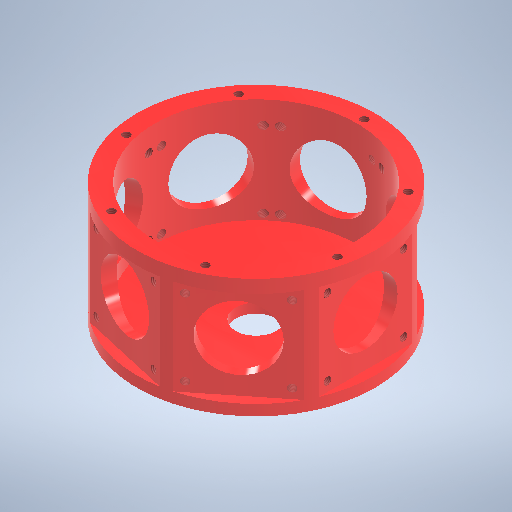
# Autodesk Inventor part: Gehäuse
Saved by Autodesk Inventor 2025 (Build 290162010, 162A)
## iProperties
Created: 2024-03-07
Part Number: Gehäuse
Material: Aluminum 6061
Document SubType Name: Modeling
Designer: ffogue
Density: 2.7 g/cm^3
Appearance: Light Red
Author: ffogue
Autodesk Inventor part; units mm, degrees
ref_plane "XZ Plane" through (0, 0, 0) normal (0, 1, 0) x (-1, 0, 0)
ref_plane "XY Plane" through (0, 0, 0) normal (0, 0, 1) x (1, 0, 0)
sketch "Skizze1" plane through (0, 0, 0) normal (0, 0, 1) x (1, 0, 0)
  circle A0 centre (0, 0) radius 50
  dimension "d0" = 100
  constraints: 1 centre point, 1 coincident
  measures "d0" diameter of A0
extrude "Extrusion1" add sketch "Skizze1" against normal blind 50
ref_plane "Arbeitsebene1" through (50, 0, 0) normal (1, 0, 0) x (0, 1, 0)
sketch "Skizze2" plane through (50, 0, 0) normal (1, 0, 0) x (0, 1, 0)
  line L0 (0, 0) -> (0, -28.5923) construction
  line L1 (-50, 0) -> (-50, -50) projected
  line L2 (-20, -5.5) -> (20, -5.5)
  line L3 (20, -5.5) -> (20, -45.5)
  line L4 (20, -45.5) -> (-20, -45.5)
  line L5 (-20, -45.5) -> (-20, -5.5)
  line L6 (-50, -50) -> (50, -50) construction
  dimension "d5" = 40
  dimension "d6" = 40
  dimension "d76" = 4.5
  constraints: 10 end point, 2 parallel, 1 horizontal, 1 perpendicular, 1 vertical, 1 other
  measures "d5" distance between parallel lines of L3 L5
  measures "d6" distance between parallel lines of L4 L2
  measures "d76" distance between parallel lines of L6 L4
extrude "Extrusion2" cut sketch "Skizze2" against normal blind 4
pattern_circular "Runde Anordnung1" count 7 over 360 about axis through (0, 0, 0) along (0, 0, -1) of "Extrusion2"
sketch "Skizze6" plane through (0, 0, -50) normal (0, 0, -1) x (-1, 0, 0)
  circle A0 centre (0, 0) radius 42.5
  circle A1 centre (0, 0) radius 40
  dimension "d25" = 85
  dimension "d26" = 80
  constraints: 2 centre point, 2 coincident
  measures "d25" diameter of A0
  measures "d26" diameter of A1
extrude "Extrusion9" cut sketch "Skizze6" against normal blind 4 contours A1
extrude "Extrusion10" add sketch "Skizze6" along normal blind 4
sketch "Sketch20" plane through (0, 0, -46) normal (0, 0, -1) x (-1, 0, 0)
  circle A0 centre (0, 0) radius 21.5
  dimension "d85" = 43
  constraints: 1 centre point, 1 coincident
  measures "d85" diameter of A0
extrude "Extrusion11" add sketch "Sketch20" along normal up to surface (8 mm away)
sketch "Sketch21" plane through (0, 0, -54) normal (0, 0, -1) x (-1, 0, 0)
  circle A0 centre (0, 0) radius 21.5 construction
  constraints: 1 coincident
hole "Hole5" at (0, 0, -54) direction (0, 0, 1) diameter 17.1 depth 4
sketch "Sketch22" plane through (0, 0, 0) normal (0, 0, 1) x (1, 0, 0)
  circle A0 centre (0, 0) radius 50 construction
  constraints: 1 coincident
hole "Hole6" at (0, 0, 0) direction (0, 0, -1) diameter 85 depth 44
sketch "Sketch24" plane through (0, 0, -50) normal (0, 0, -1) x (-1, 0, 0)
  circle A0 centre (0, 0) radius 21.5 construction
  constraints: 1 coincident
hole "Hole7" at (0, 0, -50) direction (0, 0, 1) diameter 35 depth 11
sketch "Sketch25" plane through (-32.9422, 37.614, -5.5) normal (-0.9009689, 0.4338837, 0) x (0.4338837, 0.9009689, 0)
  line L0 (0, 40) -> (-39.1918, 40) construction
  line L1 (0, 40) -> (0, 0) construction
  point P0 (-19.5959, -5.5)
  point P1 (-35.5959, 36)
  point P2 (-3.5959, 36)
  point P3 (-35.5959, 4)
  point P4 (-3.5959, 4)
  point P5 (-19.5959, 40)
  point P6 (0, 20)
  dimension "d111" = 32
  dimension "d112" = 32
  dimension "d113" = 16
  dimension "d114" = 16
  constraints: 2 horizontal alignment, 2 midpoint, 2 vertical alignment
  measures "d111" distance of point (-3.596, 36) point (-35.596, 36)
  measures "d112" distance of point (-35.596, 4) point (-35.596, 36)
  measures "d113" horizontal distance of point (-19.596, 40) point (-35.596, 36)
  measures "d114" vertical distance of point (0, 20) point (-3.596, 36)
hole "Hole8" at (-48.3867, 5.5432, -41.5) at (-34.5024, 34.3742, -41.5) at (-48.3867, 5.5432, -9.5) at (-34.5024, 34.3742, -9.5) direction (0.9009689, -0.4338837, 0) diameter 3.242 depth 10 tip angle 118 thread size "M4x0.7" class "6H" standard "ISO Metric profile"
pattern_circular "Circular Pattern4" count 7 over 360 about axis through (0, 0, -50) along (0, 0, 1) of "Hole8"
sketch "Sketch27" plane through (13.3598, -48.1821, -45.5) normal (0.6234898, -0.7818315, 0) x (0.7818315, 0.6234898, 0)
  circle A0 centre (19.5959, 21) radius 13.5
  line L0 (0, 0) -> (0, 40) construction
  line L1 (-22.9041, -8.5) -> (62.0959, -8.5) construction
  line L2 (0, 40) -> (39.1918, 40) construction
  line L3 (69.5959, 45.5) -> (-30.4041, 45.5) construction
  point P0 (19.5959, 45.5)
  point P1 (0, 20)
  point P2 (19.5959, 40)
  dimension "d132" = 27
  dimension "d153" = 24.5
  constraints: 2 midpoint, 1 centre point, 1 vertical alignment
  measures "d132" diameter of A0
  measures "d153" distance from line of L3 A0.centre
extrude "Extrusion12" cut sketch "Sketch27" against normal up to surface
pattern_circular "Circular Pattern5" count 7 over 360 about axis through (0, 0, -22) along (0, 0, 1) of "Extrusion12"
sketch "Sketch31" plane through (0, 0, -50) normal (0, 0, -1) x (-1, 0, 0)
  circle A0 centre (0, 0) radius 46 construction
  point P0 (0, 46)
  dimension "d142" = 92
  constraints: 2 vertical alignment, 1 coincident, 2 other
hole "Hole10" at (0, 46, -50) direction (0, 0, 1) diameter 4 depth 4
pattern_circular "Circular Pattern6" count 7 over 360 about axis through (0, 0, -50) along (0, 0, -1) of "Hole10"
sketch "Sketch32" plane through (0, 0, 0) normal (0, 0, 1) x (1, 0, 0)
  circle A0 centre (0, 0) radius 45.5 construction
  point P0 (0, 45.5)
  dimension "d154" = 91
  constraints: 1 coincident, 1 vertical alignment, 2 other
hole "Hole11" at (0, 45.5, 0) direction (0, 0, -1) diameter 3.242 depth 12 thread size "M4x0.7" class "6H" standard "ISO Metric profile"
pattern_circular "Circular Pattern7" count 7 over 360 about axis through (0, 0, -22) along (0, 0, 1) of "Hole11"
equation "\"d112\" = d111"
equation "\"d114\" = d113"
